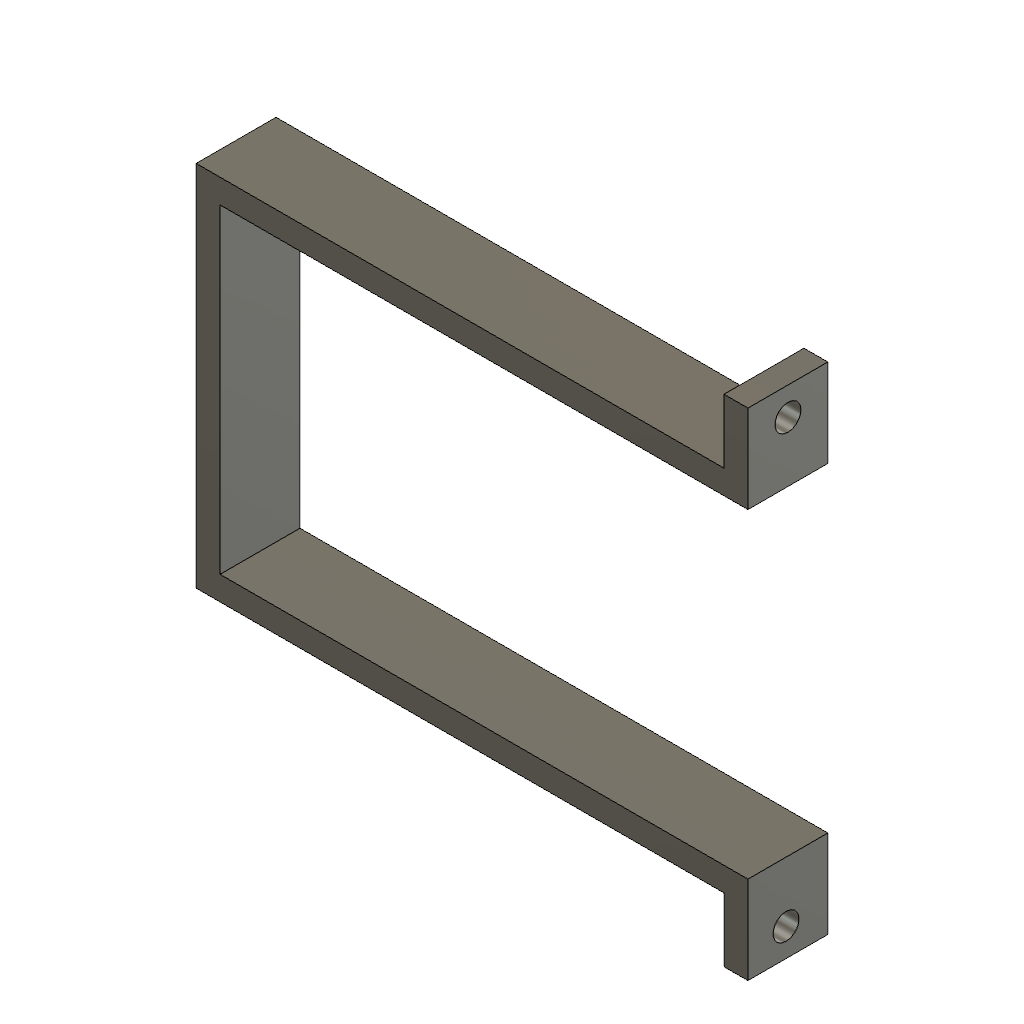
TankBot Battery Clamp (Autodesk Fusion 360 design; units mm, degrees)
Autodesk Fusion 360 part; units mm, degrees
box "BoxPrimitive1" add length 10 width 70 height 3 placed x (0, 0, 1) y (1, 0, 0) z (0, 1, 0) at (-6.409, 0, 0)
box "BoxPrimitive2" add length 10 width 3 height 40 placed x (0, 0, -1) y (-1, 0, 0) z (0, 1, 0) at (-3.409, 3, 10)
box "BoxPrimitive3" add length 10 width 70 height 3 placed x (0, 0, -1) y (-1, 0, 0) z (0, 1, 0) at (63.591, 43, 10)
box "BoxPrimitive4" add length 10 width 3 height 8 placed x (0, 0, -1) y (-1, 0, 0) z (0, 1, 0) at (63.591, 46, 10)
box "BoxPrimitive5" add length 10 width 3 height 8 placed x (0, 0, 1) y (-1, 0, 0) z (0, -1, 0) at (63.591, 0, 0)
hole "Hole1" at (60.591, -4.5, 5.237) direction (1, 0, 0) diameter 3.25 depth 3 tip angle 180
hole "Hole2" at (60.591, 50.5, 5) direction (1, 0, 0) diameter 3.25 depth 3 tip angle 180
extrude "Extrude1" add 1 faces at (-3.409, 16.3333, 3.3333) along direction (1, 0, 0) blind 1
extrude "Extrude2" cut 1 faces at (-6.409, 15.3333, 3.3333) along direction (1, 0, 0) blind 1
